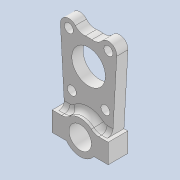
# Autodesk Inventor part: ext_conn_1
Saved by Autodesk Inventor 2020 (Build 240168000, 168)
## iProperties
Created: 2021-07-15
Part Number: ext_conn_1
Material: Generic
Document SubType Name: Modeling
Designer: Shuang Peng
Density: 1 g/cm^3
Appearance: Default
Author: Shuang Peng
Autodesk Inventor part; units mm, degrees
ref_plane "YZ Plane" through (0, 0, 0) normal (1, 0, 0) x (0, 1, 0)
ref_plane "XZ Plane" through (0, 0, 0) normal (0, 1, 0) x (-1, 0, 0)
ref_plane "XY Plane" through (0, 0, 0) normal (0, 0, 1) x (1, 0, 0)
sketch "Sketch1" plane through (0, 0, 0) normal (0, 0, 1) x (1, 0, 0)
  circle A0 centre (-3.5353, 7.9132) radius 0.8 projected
  circle A1 centre (3, -1.4962) radius 0.8 projected
  circle A2 centre (-3, -1.4962) radius 0.8 projected
  circle A3 centre (3.5353, 7.9132) radius 0.8 projected
  line L0 (-7.15, 12.3) -> (7.15, 12.3) projected
  line L1 (-7.15, 12.3) -> (-7.15, 9.7) projected
  arc A4 (-5.5752, 7.8251) -> (-7.15, 9.7) centre (-7.5736, 7.7454) ccw projected
  line L2 (-5.5752, 7.8251) -> (-4.996, -6.6992) projected
  arc A5 (-4.996, -6.6992) -> (4.996, -6.6992) centre (0, -6.5) ccw projected
  line L3 (4.996, -6.6992) -> (5.5752, 7.8251) projected
  arc A6 (7.15, 9.7) -> (5.5752, 7.8251) centre (7.5736, 7.7454) ccw projected
  line L4 (7.15, 9.7) -> (7.15, 12.3) projected
  circle A7 centre (-2.9726, -9.1765) radius 0.6 projected
  circle A8 centre (2.9726, -9.1765) radius 0.6 projected
  circle A9 centre (0, 3.7) radius 3 projected
  circle A10 centre (0, -6.5) radius 3 projected
  circle A11 centre (0, 3.7) radius 3
  line L5 (-3, -1.4962) -> (-3.5353, 7.9132) construction
  line L6 (-1.5024, -1.411) -> (-2.0378, 7.9984)
  line L7 (-5.0329, 7.828) -> (-4.4976, -1.5814)
  arc A12 (-4.4976, -1.5814) -> (-1.5024, -1.411) centre (-3, -1.4962) ccw
  arc A13 (-2.0378, 7.9984) -> (-5.0329, 7.828) centre (-3.5353, 7.9132) ccw
  line L8 (3, -1.4962) -> (3.5353, 7.9132) construction
  line L9 (4.4976, -1.5814) -> (5.0329, 7.828)
  line L10 (2.0378, 7.9984) -> (1.5024, -1.411)
  arc A14 (1.5024, -1.411) -> (4.4976, -1.5814) centre (3, -1.4962) ccw
  arc A15 (5.0329, 7.828) -> (2.0378, 7.9984) centre (3.5353, 7.9132) ccw
  circle A16 centre (0, 3.7) radius 4.5
  circle A17 centre (0, -6.5) radius 2
  line L11 (-5, -8.25) -> (-5, -4.75)
  line L12 (-5, -4.75) -> (5, -4.75)
  line L13 (5, -4.75) -> (5, -8.25)
  line L14 (5, -8.25) -> (-5, -8.25)
  line L15 (-5, -8.25) -> (5, -4.75) construction
  line L16 (-5, -4.75) -> (5, -8.25) construction
  line L17 (-4.4976, -1.5814) -> (-4.3173, -4.75)
  line L18 (4.4976, -1.5814) -> (4.3173, -4.75)
  point P0 (0, 0)
  point P1 (-3.2677, 3.2085)
  point P2 (3.2677, 3.2085)
  point P3 (2.0219, 7.7202)
  point P4 (-2.0219, 7.7202)
  point P5 (-2.4367, -8.25)
  point P6 (2.4367, -8.25)
  dimension "d0" = 6
  dimension "d1" = 3
  dimension "d2" = 3
  dimension "d3" = 9
  dimension "d4" = 4
  dimension "d5" = 3.5
  dimension "d6" = 10
  constraints: 32 end point, 8 point on circle, 8 tangent, 7 centre point, 4 midpoint, 4 parallel, 3 coincident, 3 point on line, 1 collinear, 1 perpendicular, 1 vertical
  measures "d0" diameter of A11
  measures "d1" diameter of A13
  measures "d2" diameter of A15
  measures "d3" diameter of A16
  measures "d4" diameter of A17
  measures "d5" distance of L11.start L11.end
  measures "d6" distance of L11.end L12.end
extrude "Extrusion1" add sketch "Sketch1" along normal blind 3.5 contours L11 L12 A10 L14 A5 L2 | L2 A5 L14 L11 | L13 L14 A5 L3 | L3 A5 L14 A10 L12 L13 | L17 A12 L6 A16 L10 A14 L18 L12 A10 | L14 A17 A10 | A10 L12 A17 L14 | A10 L12 A17 | L7 A13 L6 A16 A12 | L14 A17 L12 A10 | A14 L10 A16 A15 L9 | A16 L6 A9 | L6 A9 L10 A16 | L10 A9 A16 | A16 L10 A9 L6
sketch "Sketch2" plane through (0, 0, 3.5) normal (0, 0, 1) x (1, 0, 0)
  circle A0 centre (0, -6.5) radius 3 projected
  arc A1 (5.0329, 7.828) -> (2.0378, 7.9984) centre (3.5353, 7.9132) ccw projected
  line L0 (2.0378, 7.9984) -> (2.0219, 7.7202) projected
  arc A2 (2.0219, 7.7202) -> (-2.0219, 7.7202) centre (0, 3.7) ccw projected
  line L1 (-2.0219, 7.7202) -> (-2.0378, 7.9984) projected
  arc A3 (-2.0378, 7.9984) -> (-5.0329, 7.828) centre (-3.5353, 7.9132) ccw projected
  line L2 (-5.0329, 7.828) -> (-4.3173, -4.75) projected
  line L3 (-4.3173, -4.75) -> (-5, -4.75) projected
  line L4 (-5, -4.75) -> (-5, -8.25) projected
  line L5 (-5, -8.25) -> (-2.4367, -8.25) projected
  arc A4 (-2.4367, -8.25) -> (2.4367, -8.25) centre (0, -6.5) ccw projected
  line L6 (2.4367, -8.25) -> (5, -8.25) projected
  line L7 (5, -8.25) -> (5, -4.75) projected
  line L8 (5, -4.75) -> (4.3173, -4.75) projected
  line L9 (4.3173, -4.75) -> (5.0329, 7.828) projected
  circle A5 centre (0, 3.7) radius 3 projected
  circle A6 centre (0, -6.5) radius 2 projected
  circle A7 centre (3.5353, 7.9132) radius 0.8 projected
  circle A8 centre (3, -1.4962) radius 0.8 projected
  circle A9 centre (-3.5353, 7.9132) radius 0.8 projected
  circle A10 centre (-3, -1.4962) radius 0.8 projected
  line L10 (-5.0329, 7.828) -> (-4.3173, -4.75) projected
  line L11 (-4.3173, -4.75) -> (4.3173, -4.75)
  point P0 (0, 0)
  point P1 (-2.4367, -4.75)
  point P2 (2.4367, -4.75)
  constraints: 2 end point, 1 horizontal
extrude "Extrusion2" cut sketch "Sketch2" against normal blind 1.5 contours L11 L2 A3 L1 A2 L0 A1 L9 A0
fillet "Fillet1" radius 2 2 edges at (-2.0219, 7.7202, 1) (2.0219, 7.7202, 1)
sketch "Sketch3" plane through (5, -8.25, 0) normal (1, 0, 0) x (0, 0, -1)
  line L0 (0, 0) -> (0, 3.5) projected
  line L1 (0, 3.5) -> (-3.5, 3.5) projected
  line L2 (-3.5, 0) -> (-3.5, 3.5) projected
  line L3 (0, 0) -> (-3.5, 0) projected
  line L4 (-3.5, 1.75) -> (-1.75, 1.75)
  line L5 (0, 0) -> (0, 3.5) projected
  circle A0 centre (-1.75, 1.75) radius 1
  point P0 (0, 8.25)
  dimension "d14" = 1.75
  dimension "d15" = 2
  constraints: 2 end point, 1 centre point, 1 coincident, 1 midpoint, 1 perpendicular
  measures "d14" distance of L4.start L4.end
  measures "d15" diameter of A0
extrude "Extrusion3" cut sketch "Sketch3" against normal blind 10 contours A0
chamfer "Chamfer1" distance 0.5 angle 45 8 edges at (3.7183, -4.75, 3.5) (4.6587, -4.75, 0) (3.7183, -8.25, 3.5) (3.7183, -8.25, 0) (-3.7183, -4.75, 3.5) (-3.7183, -8.25, 3.5) (-4.6587, -4.75, 0) (-3.7183, -8.25, 0)
fillet "Fillet4" radius 1 4 edges at (-2.594, -4.993, 3.243) (-2.4367, -4.75, 2.5) (2.594, -4.993, 3.243) (2.4367, -4.75, 2.5)
thicken "Thicken1" operation add thickness 0.5 both sides no extend neighbours yes toward (-1, 0, 0) faces at (-5, -7.9976, 1.7098)
thicken "Thicken2" operation add thickness 0.5 both sides no extend neighbours yes toward (1, 0, 0) faces at (5, -7.9976, 1.7902)
fillet "Fillet5" radius 0.5 5 edges at (-2.5095, -4.6686, 2) (2.5095, -4.6686, 2) (3.611, -4.75, 2) (-3.611, -4.75, 2) (0, -3.5, 2)
body "Solid1"
